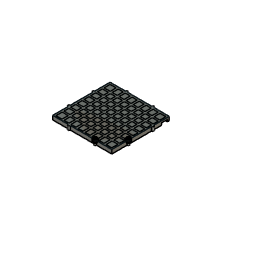
WS2812B_LED_Matrix_Diffuser (Autodesk Fusion 360 design; units mm, degrees)
Autodesk Fusion 360 part; units mm, degrees
note: some values were not read from the file. Set by a fixed rule: which face or edge a step refers to.
sketch "diffuser_base" plane through (0, 0, 0) normal (0, 0, 1) x (-1, 0, 0)
  circle A0 centre (-25.65, 24.4714) radius 1.425
  circle A1 centre (-0.15, 24.4714) radius 1.425
  circle A2 centre (25.35, 24.4714) radius 1.425
  circle A3 centre (-25.65, -24.5286) radius 1.425
  circle A4 centre (-0.15, -24.5286) radius 1.425
  circle A5 centre (25.35, -24.5286) radius 1.425
  line L0 (-33.5, -32.5) -> (-33.5, 32.5)
  line L1 (-33.5, 32.5) -> (33.5, 32.5)
  line L2 (33.5, 32.5) -> (33.5, -32.5)
  line L3 (33.5, -32.5) -> (-33.5, -32.5)
  line L4 (33.9, -32.9) -> (-33.9, -32.9)
  line L5 (-33.9, -32.9) -> (-33.9, 32.9)
  line L6 (-33.9, 32.9) -> (33.9, 32.9)
  line L7 (33.9, 32.9) -> (33.9, -32.9)
  line L8 (35.9, -34.9) -> (-35.9, -34.9)
  line L9 (-35.9, -34.9) -> (-35.9, 34.9)
  line L10 (-35.9, 34.9) -> (35.9, 34.9)
  line L11 (35.9, 34.9) -> (35.9, -34.9)
  dimension "d89" = -0.4
  dimension "d90" = -2.4
extrude "Extrude1" add sketch "diffuser_base" along normal blind 3.5 contours L8 L9 L10 L11
sketch "separations" plane through (0, 0, 1.5) normal (0, 0, 1) x (-1, 0, 0)
  circle A0 centre (25.35, 24.4714) radius 1.425
  circle A1 centre (-25.65, -24.5286) radius 1.425
  circle A2 centre (-0.15, -24.5286) radius 1.425
  circle A3 centre (25.35, -24.5286) radius 1.425
  line L0 (-27.4, 22.7571) -> (-27.4, 17.7571)
  line L1 (-27.4, 17.7571) -> (-32.4, 17.7571)
  line L2 (-32.4, 17.7571) -> (-32.4, 22.7571)
  line L3 (-32.4, 22.7571) -> (-27.4, 22.7571)
  line L4 (-18.9, 22.7571) -> (-18.9, 17.7571)
  line L5 (-18.9, 17.7571) -> (-23.9, 17.7571)
  line L6 (-23.9, 17.7571) -> (-23.9, 22.7571)
  line L7 (-23.9, 22.7571) -> (-18.9, 22.7571)
  line L8 (-10.4, 22.7571) -> (-10.4, 17.7571)
  line L9 (-10.4, 17.7571) -> (-15.4, 17.7571)
  line L10 (-15.4, 17.7571) -> (-15.4, 22.7571)
  line L11 (-15.4, 22.7571) -> (-10.4, 22.7571)
  line L12 (-1.9, 22.7571) -> (-1.9, 17.7571)
  line L13 (-1.9, 17.7571) -> (-6.9, 17.7571)
  line L14 (-6.9, 17.7571) -> (-6.9, 22.7571)
  line L15 (-6.9, 22.7571) -> (-1.9, 22.7571)
  line L16 (6.6, 22.7571) -> (6.6, 17.7571)
  line L17 (6.6, 17.7571) -> (1.6, 17.7571)
  line L18 (1.6, 17.7571) -> (1.6, 22.7571)
  line L19 (1.6, 22.7571) -> (6.6, 22.7571)
  line L20 (15.1, 22.7571) -> (15.1, 17.7571)
  line L21 (15.1, 17.7571) -> (10.1, 17.7571)
  line L22 (10.1, 17.7571) -> (10.1, 22.7571)
  line L23 (10.1, 22.7571) -> (15.1, 22.7571)
  line L24 (23.6, 22.7571) -> (23.6, 17.7571)
  line L25 (23.6, 17.7571) -> (18.6, 17.7571)
  line L26 (18.6, 17.7571) -> (18.6, 22.7571)
  line L27 (18.6, 22.7571) -> (23.6, 22.7571)
  line L28 (32.1, 22.7571) -> (32.1, 17.7571)
  line L29 (32.1, 17.7571) -> (27.1, 17.7571)
  line L30 (27.1, 17.7571) -> (27.1, 22.7571)
  line L31 (27.1, 22.7571) -> (32.1, 22.7571)
  line L32 (-27.4, 14.6143) -> (-27.4, 9.6143)
  line L33 (-27.4, 9.6143) -> (-32.4, 9.6143)
  line L34 (-32.4, 9.6143) -> (-32.4, 14.6143)
  line L35 (-32.4, 14.6143) -> (-27.4, 14.6143)
  line L36 (-18.9, 14.6143) -> (-18.9, 9.6143)
  line L37 (-18.9, 9.6143) -> (-23.9, 9.6143)
  line L38 (-23.9, 9.6143) -> (-23.9, 14.6143)
  line L39 (-23.9, 14.6143) -> (-18.9, 14.6143)
  line L40 (-10.4, 14.6143) -> (-10.4, 9.6143)
  line L41 (-10.4, 9.6143) -> (-15.4, 9.6143)
  line L42 (-15.4, 9.6143) -> (-15.4, 14.6143)
  line L43 (-15.4, 14.6143) -> (-10.4, 14.6143)
  line L44 (-1.9, 14.6143) -> (-1.9, 9.6143)
  line L45 (-1.9, 9.6143) -> (-6.9, 9.6143)
  line L46 (-6.9, 9.6143) -> (-6.9, 14.6143)
  line L47 (-6.9, 14.6143) -> (-1.9, 14.6143)
  line L48 (6.6, 14.6143) -> (6.6, 9.6143)
  line L49 (6.6, 9.6143) -> (1.6, 9.6143)
  line L50 (1.6, 9.6143) -> (1.6, 14.6143)
  line L51 (1.6, 14.6143) -> (6.6, 14.6143)
  line L52 (15.1, 14.6143) -> (15.1, 9.6143)
  line L53 (15.1, 9.6143) -> (10.1, 9.6143)
  line L54 (10.1, 9.6143) -> (10.1, 14.6143)
  line L55 (10.1, 14.6143) -> (15.1, 14.6143)
  line L56 (23.6, 14.6143) -> (23.6, 9.6143)
  line L57 (23.6, 9.6143) -> (18.6, 9.6143)
  line L58 (18.6, 9.6143) -> (18.6, 14.6143)
  line L59 (18.6, 14.6143) -> (23.6, 14.6143)
  line L60 (32.1, 14.6143) -> (32.1, 9.6143)
  line L61 (32.1, 9.6143) -> (27.1, 9.6143)
  line L62 (27.1, 9.6143) -> (27.1, 14.6143)
  line L63 (27.1, 14.6143) -> (32.1, 14.6143)
  line L64 (-27.4, 6.4714) -> (-27.4, 1.4714)
  line L65 (-27.4, 1.4714) -> (-32.4, 1.4714)
  line L66 (-32.4, 1.4714) -> (-32.4, 6.4714)
  line L67 (-32.4, 6.4714) -> (-27.4, 6.4714)
  line L68 (-18.9, 6.4714) -> (-18.9, 1.4714)
  line L69 (-18.9, 1.4714) -> (-23.9, 1.4714)
  line L70 (-23.9, 1.4714) -> (-23.9, 6.4714)
  line L71 (-23.9, 6.4714) -> (-18.9, 6.4714)
  line L72 (-10.4, 6.4714) -> (-10.4, 1.4714)
  line L73 (-10.4, 1.4714) -> (-15.4, 1.4714)
  line L74 (-15.4, 1.4714) -> (-15.4, 6.4714)
  line L75 (-15.4, 6.4714) -> (-10.4, 6.4714)
  line L76 (-1.9, 6.4714) -> (-1.9, 1.4714)
  line L77 (-1.9, 1.4714) -> (-6.9, 1.4714)
  line L78 (-6.9, 1.4714) -> (-6.9, 6.4714)
  line L79 (-6.9, 6.4714) -> (-1.9, 6.4714)
  line L80 (6.6, 6.4714) -> (6.6, 1.4714)
  line L81 (6.6, 1.4714) -> (1.6, 1.4714)
  line L82 (1.6, 1.4714) -> (1.6, 6.4714)
  line L83 (1.6, 6.4714) -> (6.6, 6.4714)
  line L84 (15.1, 6.4714) -> (15.1, 1.4714)
  line L85 (15.1, 1.4714) -> (10.1, 1.4714)
  line L86 (10.1, 1.4714) -> (10.1, 6.4714)
  line L87 (10.1, 6.4714) -> (15.1, 6.4714)
  line L88 (23.6, 6.4714) -> (23.6, 1.4714)
  line L89 (23.6, 1.4714) -> (18.6, 1.4714)
  line L90 (18.6, 1.4714) -> (18.6, 6.4714)
  line L91 (18.6, 6.4714) -> (23.6, 6.4714)
  line L92 (32.1, 6.4714) -> (32.1, 1.4714)
  line L93 (32.1, 1.4714) -> (27.1, 1.4714)
  line L94 (27.1, 1.4714) -> (27.1, 6.4714)
  line L95 (27.1, 6.4714) -> (32.1, 6.4714)
  line L96 (-27.4, -1.6714) -> (-27.4, -6.6714)
  line L97 (-27.4, -6.6714) -> (-32.4, -6.6714)
  line L98 (-32.4, -6.6714) -> (-32.4, -1.6714)
  line L99 (-32.4, -1.6714) -> (-27.4, -1.6714)
  line L100 (-18.9, -1.6714) -> (-18.9, -6.6714)
  line L101 (-18.9, -6.6714) -> (-23.9, -6.6714)
  line L102 (-23.9, -6.6714) -> (-23.9, -1.6714)
  line L103 (-23.9, -1.6714) -> (-18.9, -1.6714)
  line L104 (-10.4, -1.6714) -> (-10.4, -6.6714)
  line L105 (-10.4, -6.6714) -> (-15.4, -6.6714)
  line L106 (-15.4, -6.6714) -> (-15.4, -1.6714)
  line L107 (-15.4, -1.6714) -> (-10.4, -1.6714)
  line L108 (-1.9, -1.6714) -> (-1.9, -6.6714)
  line L109 (-1.9, -6.6714) -> (-6.9, -6.6714)
  line L110 (-6.9, -6.6714) -> (-6.9, -1.6714)
  line L111 (-6.9, -1.6714) -> (-1.9, -1.6714)
  line L112 (6.6, -1.6714) -> (6.6, -6.6714)
  line L113 (6.6, -6.6714) -> (1.6, -6.6714)
  line L114 (1.6, -6.6714) -> (1.6, -1.6714)
  line L115 (1.6, -1.6714) -> (6.6, -1.6714)
  line L116 (15.1, -1.6714) -> (15.1, -6.6714)
  line L117 (15.1, -6.6714) -> (10.1, -6.6714)
  line L118 (10.1, -6.6714) -> (10.1, -1.6714)
  line L119 (10.1, -1.6714) -> (15.1, -1.6714)
  line L120 (23.6, -1.6714) -> (23.6, -6.6714)
  line L121 (23.6, -6.6714) -> (18.6, -6.6714)
  line L122 (18.6, -6.6714) -> (18.6, -1.6714)
  line L123 (18.6, -1.6714) -> (23.6, -1.6714)
  line L124 (32.1, -1.6714) -> (32.1, -6.6714)
  line L125 (32.1, -6.6714) -> (27.1, -6.6714)
  line L126 (27.1, -6.6714) -> (27.1, -1.6714)
  line L127 (27.1, -1.6714) -> (32.1, -1.6714)
  line L128 (-27.4, -9.8143) -> (-27.4, -14.8143)
  line L129 (-27.4, -14.8143) -> (-32.4, -14.8143)
  line L130 (-32.4, -14.8143) -> (-32.4, -9.8143)
  line L131 (-32.4, -9.8143) -> (-27.4, -9.8143)
  line L132 (-18.9, -9.8143) -> (-18.9, -14.8143)
  line L133 (-18.9, -14.8143) -> (-23.9, -14.8143)
  line L134 (-23.9, -14.8143) -> (-23.9, -9.8143)
  line L135 (-23.9, -9.8143) -> (-18.9, -9.8143)
  line L136 (-10.4, -9.8143) -> (-10.4, -14.8143)
  line L137 (-10.4, -14.8143) -> (-15.4, -14.8143)
  line L138 (-15.4, -14.8143) -> (-15.4, -9.8143)
  line L139 (-15.4, -9.8143) -> (-10.4, -9.8143)
  line L140 (-1.9, -9.8143) -> (-1.9, -14.8143)
  line L141 (-1.9, -14.8143) -> (-6.9, -14.8143)
  line L142 (-6.9, -14.8143) -> (-6.9, -9.8143)
  line L143 (-6.9, -9.8143) -> (-1.9, -9.8143)
  line L144 (6.6, -9.8143) -> (6.6, -14.8143)
  line L145 (6.6, -14.8143) -> (1.6, -14.8143)
  line L146 (1.6, -14.8143) -> (1.6, -9.8143)
  line L147 (1.6, -9.8143) -> (6.6, -9.8143)
  line L148 (15.1, -9.8143) -> (15.1, -14.8143)
  line L149 (15.1, -14.8143) -> (10.1, -14.8143)
  line L150 (10.1, -14.8143) -> (10.1, -9.8143)
  line L151 (10.1, -9.8143) -> (15.1, -9.8143)
  line L152 (23.6, -9.8143) -> (23.6, -14.8143)
  line L153 (23.6, -14.8143) -> (18.6, -14.8143)
  line L154 (18.6, -14.8143) -> (18.6, -9.8143)
  line L155 (18.6, -9.8143) -> (23.6, -9.8143)
  line L156 (32.1, -9.8143) -> (32.1, -14.8143)
  line L157 (32.1, -14.8143) -> (27.1, -14.8143)
  line L158 (27.1, -14.8143) -> (27.1, -9.8143)
  line L159 (27.1, -9.8143) -> (32.1, -9.8143)
  line L160 (-27.4, -17.9571) -> (-27.4, -22.9571)
  line L161 (-27.4, -22.9571) -> (-32.4, -22.9571)
  line L162 (-32.4, -22.9571) -> (-32.4, -17.9571)
  line L163 (-32.4, -17.9571) -> (-27.4, -17.9571)
  line L164 (-18.9, -17.9571) -> (-18.9, -22.9571)
  line L165 (-18.9, -22.9571) -> (-23.9, -22.9571)
  line L166 (-23.9, -22.9571) -> (-23.9, -17.9571)
  line L167 (-23.9, -17.9571) -> (-18.9, -17.9571)
  line L168 (-10.4, -17.9571) -> (-10.4, -22.9571)
  line L169 (-10.4, -22.9571) -> (-15.4, -22.9571)
  line L170 (-15.4, -22.9571) -> (-15.4, -17.9571)
  line L171 (-15.4, -17.9571) -> (-10.4, -17.9571)
  line L172 (-1.9, -17.9571) -> (-1.9, -22.9571)
  line L173 (-1.9, -22.9571) -> (-6.9, -22.9571)
  line L174 (-6.9, -22.9571) -> (-6.9, -17.9571)
  line L175 (-6.9, -17.9571) -> (-1.9, -17.9571)
  line L176 (6.6, -17.9571) -> (6.6, -22.9571)
  line L177 (6.6, -22.9571) -> (1.6, -22.9571)
  line L178 (1.6, -22.9571) -> (1.6, -17.9571)
  line L179 (1.6, -17.9571) -> (6.6, -17.9571)
  line L180 (15.1, -17.9571) -> (15.1, -22.9571)
  line L181 (15.1, -22.9571) -> (10.1, -22.9571)
  line L182 (10.1, -22.9571) -> (10.1, -17.9571)
  line L183 (10.1, -17.9571) -> (15.1, -17.9571)
  line L184 (23.6, -17.9571) -> (23.6, -22.9571)
  line L185 (23.6, -22.9571) -> (18.6, -22.9571)
  line L186 (18.6, -22.9571) -> (18.6, -17.9571)
  line L187 (18.6, -17.9571) -> (23.6, -17.9571)
  line L188 (32.1, -17.9571) -> (32.1, -22.9571)
  line L189 (32.1, -22.9571) -> (27.1, -22.9571)
  line L190 (27.1, -22.9571) -> (27.1, -17.9571)
  line L191 (27.1, -17.9571) -> (32.1, -17.9571)
  line L192 (-27.4, -26.1) -> (-27.4, -31.1)
  line L193 (-27.4, -31.1) -> (-32.4, -31.1)
  line L194 (-32.4, -31.1) -> (-32.4, -26.1)
  line L195 (-32.4, -26.1) -> (-27.4, -26.1)
  line L196 (-18.9, -26.1) -> (-18.9, -31.1)
  line L197 (-18.9, -31.1) -> (-23.9, -31.1)
  line L198 (-23.9, -31.1) -> (-23.9, -26.1)
  line L199 (-23.9, -26.1) -> (-18.9, -26.1)
  line L200 (-10.4, -26.1) -> (-10.4, -31.1)
  line L201 (-10.4, -31.1) -> (-15.4, -31.1)
  line L202 (-15.4, -31.1) -> (-15.4, -26.1)
  line L203 (-15.4, -26.1) -> (-10.4, -26.1)
  line L204 (-1.9, -26.1) -> (-1.9, -31.1)
  line L205 (-1.9, -31.1) -> (-6.9, -31.1)
  line L206 (-6.9, -31.1) -> (-6.9, -26.1)
  line L207 (-6.9, -26.1) -> (-1.9, -26.1)
  line L208 (6.6, -26.1) -> (6.6, -31.1)
  line L209 (6.6, -31.1) -> (1.6, -31.1)
  line L210 (1.6, -31.1) -> (1.6, -26.1)
  line L211 (1.6, -26.1) -> (6.6, -26.1)
  line L212 (15.1, -26.1) -> (15.1, -31.1)
  line L213 (15.1, -31.1) -> (10.1, -31.1)
  line L214 (10.1, -31.1) -> (10.1, -26.1)
  line L215 (10.1, -26.1) -> (15.1, -26.1)
  line L216 (23.6, -26.1) -> (23.6, -31.1)
  line L217 (23.6, -31.1) -> (18.6, -31.1)
  line L218 (18.6, -31.1) -> (18.6, -26.1)
  line L219 (18.6, -26.1) -> (23.6, -26.1)
  line L220 (32.1, -26.1) -> (32.1, -31.1)
  line L221 (32.1, -31.1) -> (27.1, -31.1)
  line L222 (27.1, -31.1) -> (27.1, -26.1)
  line L223 (27.1, -26.1) -> (32.1, -26.1)
  line L224 (-33.5, 32.5) -> (-33.5, -32.5)
  line L225 (-33.5, -32.5) -> (33.5, -32.5)
  line L226 (33.5, -32.5) -> (33.5, 32.5)
  line L227 (33.5, 32.5) -> (-33.5, 32.5)
  line L228 (-27.4, -26.1) -> (-32.4, -26.1)
  line L229 (-32.4, -22.9571) -> (-27.4, -22.9571)
  line L230 (33.9, -25.6) -> (-33.9, -25.6)
  line L231 (-33.9, -25.6) -> (-33.9, -23.4571)
  line L232 (-33.9, -23.4571) -> (33.9, -23.4571)
  line L233 (33.9, -23.4571) -> (33.9, -25.6)
  line L234 (-23.9, -26.1) -> (-23.9, -31.1)
  line L235 (-27.4, -31.1) -> (-27.4, -26.1)
  line L236 (-24.4, -32.9) -> (-26.9, -32.9)
  line L237 (-26.9, -32.9) -> (-26.9, 32.9)
  line L238 (-26.9, 32.9) -> (-24.4, 32.9)
  line L239 (-24.4, 32.9) -> (-24.4, -32.9)
  circle A4 centre (-25.65, 24.4714) radius 1.425
  circle A5 centre (-0.15, 24.4714) radius 1.425
  line L240 (-27.4, 30.9) -> (-27.4, 25.9)
  line L241 (-27.4, 25.9) -> (-32.4, 25.9)
  line L242 (-32.4, 25.9) -> (-32.4, 30.9)
  line L243 (-32.4, 30.9) -> (-27.4, 30.9)
  line L244 (-18.9, 30.9) -> (-18.9, 25.9)
  line L245 (-18.9, 25.9) -> (-23.9, 25.9)
  line L246 (-23.9, 25.9) -> (-23.9, 30.9)
  line L247 (-23.9, 30.9) -> (-18.9, 30.9)
  line L248 (-10.4, 30.9) -> (-10.4, 25.9)
  line L249 (-10.4, 25.9) -> (-15.4, 25.9)
  line L250 (-15.4, 25.9) -> (-15.4, 30.9)
  line L251 (-15.4, 30.9) -> (-10.4, 30.9)
  line L252 (-1.9, 30.9) -> (-1.9, 25.9)
  line L253 (-1.9, 25.9) -> (-6.9, 25.9)
  line L254 (-6.9, 25.9) -> (-6.9, 30.9)
  line L255 (-6.9, 30.9) -> (-1.9, 30.9)
  line L256 (6.6, 30.9) -> (6.6, 25.9)
  line L257 (6.6, 25.9) -> (1.6, 25.9)
  line L258 (1.6, 25.9) -> (1.6, 30.9)
  line L259 (1.6, 30.9) -> (6.6, 30.9)
  line L260 (15.1, 30.9) -> (15.1, 25.9)
  line L261 (15.1, 25.9) -> (10.1, 25.9)
  line L262 (10.1, 25.9) -> (10.1, 30.9)
  line L263 (10.1, 30.9) -> (15.1, 30.9)
  line L264 (23.6, 30.9) -> (23.6, 25.9)
  line L265 (23.6, 25.9) -> (18.6, 25.9)
  line L266 (18.6, 25.9) -> (18.6, 30.9)
  line L267 (18.6, 30.9) -> (23.6, 30.9)
  line L268 (32.1, 30.9) -> (32.1, 25.9)
  line L269 (32.1, 25.9) -> (27.1, 25.9)
  line L270 (27.1, 25.9) -> (27.1, 30.9)
  line L271 (27.1, 30.9) -> (32.1, 30.9)
  line L272 (33.9, 32.9) -> (33.9, -32.9)
  line L273 (33.9, -32.9) -> (-33.9, -32.9)
  line L274 (-33.9, -32.9) -> (-33.9, 32.9)
  line L275 (-33.9, 32.9) -> (33.9, 32.9)
  dimension "d26" = 0.5
  dimension "d27" = 0.5
  dimension "d28" = 0.5
  dimension "d29" = 0.5
  constraint horizontal L230
  constraint vertical L231
  constraint horizontal L232
  constraint vertical L233
  constraint horizontal L236
  constraint vertical L237
  constraint horizontal L238
  constraint vertical L239
  constraint collinear L233 L272
  constraint collinear L231 L274
  constraint collinear L236 L273
  constraint collinear L238 L275
  measures "d26" distance of L228 L230
  measures "d27" distance of L229 L232
  measures "d28" distance of L234 L239
  measures "d29" distance of L235 L237
extrude "Extrude2" add sketch "separations" along normal blind 2 contours A1 L230 L232 L237 L239 | A1 L232 L239 | A1 L230 L239 | A1 L232 | A1 L232 L237 L239 A4 | A1 L225 L230 L237 L239 | A1 L230 | A1 L232 L237 | L237 L239 A4 | A1 L230 L237 | L225 L236 L237 L239 L273 | L227 L237 L239 A4 | L227 L237 L238 L239 L275
extrude "Extrude3" add sketch "separations" along normal blind 2 contours A1 L239 | A1 A2 L230 L232 L239 | A2 L230 L232 | A1 L237 | A1 L224 L230 L232 L237 | A2 A3 L230 L232 | L224 L230 L231 L232 L274 | A3 L230 L232 | A3 L226 L230 L232 | L226 L230 L232 L233 L272
pattern_linear "R-Pattern1" count 7 spacing 8.5 along (-1, 0, 0) of "Extrude2"
pattern_linear "R-Pattern2" count 7 spacing 8.15 along (0, -1, 0) of "Extrude3"
sketch "cover" plane through (0, 0, 3.5) normal (0, 0, 1) x (-1, 0, 0)
  line L0 (-26.9, 32.9) -> (-26.9, 25.4429)
  line L1 (-26.9, 25.4429) -> (-33.9, 25.4429)
  line L2 (33.9, 17.2929) -> (26.6, 17.2929)
  line L3 (26.6, 17.2929) -> (26.6, 23.3)
  line L4 (26.6, 23.3) -> (33.9, 23.3)
  line L5 (18.1, 25.4429) -> (18.1, 32.9)
  line L6 (24.1, 32.9) -> (24.1, 25.4429)
  line L7 (24.1, 25.4429) -> (18.1, 25.4429)
  line L8 (15.6, 23.3) -> (15.6, 17.2929)
  line L9 (15.6, 17.2929) -> (9.6, 17.2929)
  line L10 (9.6, 17.2929) -> (9.6, 23.3)
  line L11 (9.6, 23.3) -> (15.6, 23.3)
  line L12 (7.1, 23.3) -> (7.1, 17.2929)
  line L13 (7.1, 17.2929) -> (1.1, 17.2929)
  line L14 (1.1, 17.2929) -> (1.1, 23.3)
  line L15 (1.1, 23.3) -> (7.1, 23.3)
  line L16 (-1.4, 23.3) -> (-1.4, 17.2929)
  line L17 (-1.4, 17.2929) -> (-7.4, 17.2929)
  line L18 (-7.4, 17.2929) -> (-7.4, 23.3)
  line L19 (-7.4, 23.3) -> (-1.4, 23.3)
  line L20 (-9.9, 23.3) -> (-9.9, 17.2929)
  line L21 (-9.9, 17.2929) -> (-15.9, 17.2929)
  line L22 (-15.9, 17.2929) -> (-15.9, 23.3)
  line L23 (-15.9, 23.3) -> (-9.9, 23.3)
  line L24 (-18.4, 23.3) -> (-18.4, 17.2929)
  line L25 (-18.4, 17.2929) -> (-24.4, 17.2929)
  line L26 (-24.4, 17.2929) -> (-24.4, 23.3)
  line L27 (-24.4, 23.3) -> (-18.4, 23.3)
  line L28 (18.1, 23.3) -> (24.1, 23.3)
  line L29 (24.1, 23.3) -> (24.1, 17.2929)
  line L30 (24.1, 17.2929) -> (18.1, 17.2929)
  line L31 (18.1, 17.2929) -> (18.1, 23.3)
  line L32 (15.6, 25.4429) -> (9.6, 25.4429)
  line L33 (9.6, 25.4429) -> (9.6, 32.9)
  line L34 (7.1, 25.4429) -> (1.1, 25.4429)
  line L35 (1.1, 25.4429) -> (1.1, 32.9)
  line L36 (-1.4, 25.4429) -> (-7.4, 25.4429)
  line L37 (-7.4, 25.4429) -> (-7.4, 32.9)
  line L38 (-9.9, 25.4429) -> (-15.9, 25.4429)
  line L39 (-15.9, 25.4429) -> (-15.9, 32.9)
  line L40 (26.6, 25.4429) -> (26.6, 32.9)
  line L41 (-18.4, 25.4429) -> (-24.4, 25.4429)
  line L42 (-24.4, 25.4429) -> (-24.4, 32.9)
  line L43 (-33.9, 23.3) -> (-26.9, 23.3)
  line L44 (-26.9, 23.3) -> (-26.9, 17.2929)
  line L45 (-26.9, 17.2929) -> (-33.9, 17.2929)
  line L46 (33.9, 9.1429) -> (26.6, 9.1429)
  line L47 (26.6, 9.1429) -> (26.6, 15.15)
  line L48 (26.6, 15.15) -> (33.9, 15.15)
  line L49 (24.1, 15.15) -> (24.1, 9.1429)
  line L50 (24.1, 9.1429) -> (18.1, 9.1429)
  line L51 (18.1, 9.1429) -> (18.1, 15.15)
  line L52 (18.1, 15.15) -> (24.1, 15.15)
  line L53 (15.6, 15.15) -> (15.6, 9.1429)
  line L54 (15.6, 9.1429) -> (9.6, 9.1429)
  line L55 (9.6, 9.1429) -> (9.6, 15.15)
  line L56 (9.6, 15.15) -> (15.6, 15.15)
  line L57 (7.1, 15.15) -> (7.1, 9.1429)
  line L58 (7.1, 9.1429) -> (1.1, 9.1429)
  line L59 (1.1, 9.1429) -> (1.1, 15.15)
  line L60 (1.1, 15.15) -> (7.1, 15.15)
  line L61 (-1.4, 15.15) -> (-1.4, 9.1429)
  line L62 (-1.4, 9.1429) -> (-7.4, 9.1429)
  line L63 (-7.4, 9.1429) -> (-7.4, 15.15)
  line L64 (-7.4, 15.15) -> (-1.4, 15.15)
  line L65 (-9.9, 15.15) -> (-9.9, 9.1429)
  line L66 (-9.9, 9.1429) -> (-15.9, 9.1429)
  line L67 (-15.9, 9.1429) -> (-15.9, 15.15)
  line L68 (-15.9, 15.15) -> (-9.9, 15.15)
  line L69 (-18.4, 15.15) -> (-18.4, 9.1429)
  line L70 (-18.4, 9.1429) -> (-24.4, 9.1429)
  line L71 (-24.4, 9.1429) -> (-24.4, 15.15)
  line L72 (-24.4, 15.15) -> (-18.4, 15.15)
  line L73 (-33.9, 7) -> (-26.9, 7)
  line L74 (-26.9, 7) -> (-26.9, 0.9929)
  line L75 (-26.9, 0.9929) -> (-33.9, 0.9929)
  line L76 (33.9, -7.1571) -> (26.6, -7.1571)
  line L77 (26.6, -7.1571) -> (26.6, -1.15)
  line L78 (26.6, -1.15) -> (33.9, -1.15)
  line L79 (24.1, -1.15) -> (24.1, -7.1571)
  line L80 (24.1, -7.1571) -> (18.1, -7.1571)
  line L81 (18.1, -7.1571) -> (18.1, -1.15)
  line L82 (18.1, -1.15) -> (24.1, -1.15)
  line L83 (-18.4, -1.15) -> (-18.4, -7.1571)
  line L84 (-18.4, -7.1571) -> (-24.4, -7.1571)
  line L85 (-24.4, -7.1571) -> (-24.4, -1.15)
  line L86 (-24.4, -1.15) -> (-18.4, -1.15)
  line L87 (-15.9, -1.15) -> (-9.9, -1.15)
  line L88 (-9.9, -1.15) -> (-9.9, -7.1571)
  line L89 (-9.9, -7.1571) -> (-15.9, -7.1571)
  line L90 (-15.9, -7.1571) -> (-15.9, -1.15)
  line L91 (-7.4, -1.15) -> (-1.4, -1.15)
  line L92 (-1.4, -1.15) -> (-1.4, -7.1571)
  line L93 (-1.4, -7.1571) -> (-7.4, -7.1571)
  line L94 (-7.4, -7.1571) -> (-7.4, -1.15)
  line L95 (1.1, -1.15) -> (7.1, -1.15)
  line L96 (7.1, -1.15) -> (7.1, -7.1571)
  line L97 (7.1, -7.1571) -> (1.1, -7.1571)
  line L98 (1.1, -7.1571) -> (1.1, -1.15)
  line L99 (9.6, -1.15) -> (15.6, -1.15)
  line L100 (15.6, -1.15) -> (15.6, -7.1571)
  line L101 (15.6, -7.1571) -> (9.6, -7.1571)
  line L102 (9.6, -7.1571) -> (9.6, -1.15)
  line L103 (-33.9, -1.15) -> (-26.9, -1.15)
  line L104 (-26.9, -1.15) -> (-26.9, -7.1571)
  line L105 (-26.9, -7.1571) -> (-33.9, -7.1571)
  line L106 (33.9, -15.3071) -> (26.6, -15.3071)
  line L107 (26.6, -15.3071) -> (26.6, -9.3)
  line L108 (26.6, -9.3) -> (33.9, -9.3)
  line L109 (7.1, -9.3) -> (7.1, -15.3071)
  line L110 (7.1, -15.3071) -> (1.1, -15.3071)
  line L111 (1.1, -15.3071) -> (1.1, -9.3)
  line L112 (1.1, -9.3) -> (7.1, -9.3)
  line L113 (-1.4, -9.3) -> (-1.4, -15.3071)
  line L114 (-1.4, -15.3071) -> (-7.4, -15.3071)
  line L115 (-7.4, -15.3071) -> (-7.4, -9.3)
  line L116 (-7.4, -9.3) -> (-1.4, -9.3)
  line L117 (-18.4, -9.3) -> (-18.4, -15.3071)
  line L118 (-18.4, -15.3071) -> (-24.4, -15.3071)
  line L119 (-24.4, -15.3071) -> (-24.4, -9.3)
  line L120 (-24.4, -9.3) -> (-18.4, -9.3)
  line L121 (24.1, -9.3) -> (24.1, -15.3071)
  line L122 (24.1, -15.3071) -> (18.1, -15.3071)
  line L123 (18.1, -15.3071) -> (18.1, -9.3)
  line L124 (18.1, -9.3) -> (24.1, -9.3)
  line L125 (9.6, -9.3) -> (15.6, -9.3)
  line L126 (15.6, -9.3) -> (15.6, -15.3071)
  line L127 (15.6, -15.3071) -> (9.6, -15.3071)
  line L128 (9.6, -15.3071) -> (9.6, -9.3)
  line L129 (-15.9, -9.3) -> (-9.9, -9.3)
  line L130 (-9.9, -9.3) -> (-9.9, -15.3071)
  line L131 (-9.9, -15.3071) -> (-15.9, -15.3071)
  line L132 (-15.9, -15.3071) -> (-15.9, -9.3)
  line L133 (-33.9, -9.3) -> (-26.9, -9.3)
  line L134 (-26.9, -9.3) -> (-26.9, -15.3071)
  line L135 (-26.9, -15.3071) -> (-33.9, -15.3071)
  line L136 (33.9, -23.4571) -> (26.6, -23.4571)
  line L137 (26.6, -23.4571) -> (26.6, -17.45)
  line L138 (26.6, -17.45) -> (33.9, -17.45)
  line L139 (24.1, -17.45) -> (24.1, -23.4571)
  line L140 (24.1, -23.4571) -> (18.1, -23.4571)
  line L141 (18.1, -23.4571) -> (18.1, -17.45)
  line L142 (18.1, -17.45) -> (24.1, -17.45)
  line L143 (15.6, -17.45) -> (15.6, -23.4571)
  line L144 (15.6, -23.4571) -> (9.6, -23.4571)
  line L145 (9.6, -23.4571) -> (9.6, -17.45)
  line L146 (9.6, -17.45) -> (15.6, -17.45)
  line L147 (7.1, -17.45) -> (7.1, -23.4571)
  line L148 (7.1, -23.4571) -> (1.1, -23.4571)
  line L149 (1.1, -23.4571) -> (1.1, -17.45)
  line L150 (1.1, -17.45) -> (7.1, -17.45)
  line L151 (-1.4, -17.45) -> (-1.4, -23.4571)
  line L152 (-1.4, -23.4571) -> (-7.4, -23.4571)
  line L153 (-7.4, -23.4571) -> (-7.4, -17.45)
  line L154 (-7.4, -17.45) -> (-1.4, -17.45)
  line L155 (-18.4, -17.45) -> (-18.4, -23.4571)
  line L156 (-18.4, -23.4571) -> (-24.4, -23.4571)
  line L157 (-24.4, -23.4571) -> (-24.4, -17.45)
  line L158 (-24.4, -17.45) -> (-18.4, -17.45)
  line L159 (-15.9, -17.45) -> (-9.9, -17.45)
  line L160 (-9.9, -17.45) -> (-9.9, -23.4571)
  line L161 (-9.9, -23.4571) -> (-15.9, -23.4571)
  line L162 (-15.9, -23.4571) -> (-15.9, -17.45)
  line L163 (1.1, -25.6) -> (7.1, -25.6)
  line L164 (7.1, -25.6) -> (7.1, -32.9)
  line L165 (-7.4, -25.6) -> (-1.4, -25.6)
  line L166 (-1.4, -25.6) -> (-1.4, -32.9)
  line L167 (-15.9, -25.6) -> (-9.9, -25.6)
  line L168 (-9.9, -25.6) -> (-9.9, -32.9)
  line L169 (-24.4, -25.6) -> (-18.4, -25.6)
  line L170 (-18.4, -25.6) -> (-18.4, -32.9)
  line L171 (-33.9, -25.6) -> (-26.9, -25.6)
  line L172 (-26.9, -25.6) -> (-26.9, -32.9)
  line L173 (-33.9, -17.45) -> (-26.9, -17.45)
  line L174 (-26.9, -17.45) -> (-26.9, -23.4571)
  line L175 (-26.9, -23.4571) -> (-33.9, -23.4571)
  line L176 (9.6, -25.6) -> (15.6, -25.6)
  line L177 (15.6, -25.6) -> (15.6, -32.9)
  line L178 (26.6, -25.6) -> (33.9, -25.6)
  line L179 (18.1, -25.6) -> (24.1, -25.6)
  line L180 (24.1, -25.6) -> (24.1, -32.9)
  line L181 (18.1, 7) -> (24.1, 7)
  line L182 (24.1, 7) -> (24.1, 0.9929)
  line L183 (24.1, 0.9929) -> (18.1, 0.9929)
  line L184 (18.1, 0.9929) -> (18.1, 7)
  line L185 (9.6, 7) -> (15.6, 7)
  line L186 (15.6, 7) -> (15.6, 0.9929)
  line L187 (15.6, 0.9929) -> (9.6, 0.9929)
  line L188 (9.6, 0.9929) -> (9.6, 7)
  line L189 (1.1, 7) -> (7.1, 7)
  line L190 (7.1, 7) -> (7.1, 0.9929)
  line L191 (7.1, 0.9929) -> (1.1, 0.9929)
  line L192 (1.1, 0.9929) -> (1.1, 7)
  line L193 (-7.4, 7) -> (-1.4, 7)
  line L194 (-1.4, 7) -> (-1.4, 0.9929)
  line L195 (-1.4, 0.9929) -> (-7.4, 0.9929)
  line L196 (-7.4, 0.9929) -> (-7.4, 7)
  line L197 (-15.9, 7) -> (-9.9, 7)
  line L198 (-9.9, 7) -> (-9.9, 0.9929)
  line L199 (-9.9, 0.9929) -> (-15.9, 0.9929)
  line L200 (-15.9, 0.9929) -> (-15.9, 7)
  line L201 (-18.4, 7) -> (-18.4, 0.9929)
  line L202 (-18.4, 0.9929) -> (-24.4, 0.9929)
  line L203 (-24.4, 0.9929) -> (-24.4, 7)
  line L204 (-24.4, 7) -> (-18.4, 7)
  line L205 (26.6, 0.9929) -> (26.6, 7)
  line L206 (26.6, 7) -> (33.9, 7)
  line L207 (-33.9, 15.15) -> (-26.9, 15.15)
  line L208 (-26.9, 15.15) -> (-26.9, 9.1429)
  line L209 (-26.9, 9.1429) -> (-33.9, 9.1429)
  circle A0 centre (25.35, -24.5286) radius 1.425
  circle A1 centre (-0.15, -24.5286) radius 1.425
  circle A2 centre (-25.65, -24.5286) radius 1.425
  circle A3 centre (25.35, 24.4714) radius 1.425
  circle A4 centre (-0.15, 24.4714) radius 1.425
  circle A5 centre (-25.65, 24.4714) radius 1.425
  line L210 (18.1, 32.9) -> (24.1, 32.9)
  line L211 (9.6, 32.9) -> (15.6, 32.9)
  line L212 (15.6, 32.9) -> (15.6, 25.4429)
  line L213 (1.1, 32.9) -> (7.1, 32.9)
  line L214 (7.1, 32.9) -> (7.1, 25.4429)
  line L215 (-7.4, 32.9) -> (-1.4, 32.9)
  line L216 (-1.4, 32.9) -> (-1.4, 25.4429)
  line L217 (-15.9, 32.9) -> (-9.9, 32.9)
  line L218 (-9.9, 32.9) -> (-9.9, 25.4429)
  line L219 (26.6, 32.9) -> (33.9, 32.9)
  line L220 (33.9, 23.3) -> (33.9, 17.2929)
  line L221 (33.9, -32.9) -> (26.6, -32.9)
  line L222 (-24.4, 32.9) -> (-18.4, 32.9)
  line L223 (-18.4, 32.9) -> (-18.4, 25.4429)
  line L224 (15.6, -32.9) -> (9.6, -32.9)
  line L225 (9.6, -32.9) -> (9.6, -25.6)
  line L226 (-1.4, -32.9) -> (-7.4, -32.9)
  line L227 (-7.4, -32.9) -> (-7.4, -25.6)
  line L228 (-18.4, -32.9) -> (-24.4, -32.9)
  line L229 (-24.4, -32.9) -> (-24.4, -25.6)
  line L230 (35.9, 34.9) -> (-35.9, 34.9)
  line L231 (-35.9, 34.9) -> (-35.9, -34.9)
  line L232 (-35.9, -34.9) -> (35.9, -34.9)
  line L233 (35.9, -34.9) -> (35.9, 34.9)
  line L234 (-26.9, -32.9) -> (-33.9, -32.9)
  line L235 (-33.9, 25.4429) -> (-33.9, 32.9)
  line L236 (-33.9, 32.9) -> (-26.9, 32.9)
  line L237 (-9.9, -32.9) -> (-15.9, -32.9)
  line L238 (-15.9, -32.9) -> (-15.9, -25.6)
  line L239 (7.1, -32.9) -> (1.1, -32.9)
  line L240 (1.1, -32.9) -> (1.1, -25.6)
  line L241 (24.1, -32.9) -> (18.1, -32.9)
  line L242 (18.1, -32.9) -> (18.1, -25.6)
  line L243 (33.9, 25.4429) -> (26.6, 25.4429)
  line L244 (33.9, 32.9) -> (33.9, 25.4429)
  line L245 (-33.9, 17.2929) -> (-33.9, 23.3)
  line L246 (33.9, 15.15) -> (33.9, 9.1429)
  line L247 (-33.9, 0.9929) -> (-33.9, 7)
  line L248 (33.9, -1.15) -> (33.9, -7.1571)
  line L249 (-33.9, -7.1571) -> (-33.9, -1.15)
  line L250 (33.9, -9.3) -> (33.9, -15.3071)
  line L251 (-33.9, -15.3071) -> (-33.9, -9.3)
  line L252 (33.9, -17.45) -> (33.9, -23.4571)
  line L253 (-33.9, -32.9) -> (-33.9, -25.6)
  line L254 (-33.9, -23.4571) -> (-33.9, -17.45)
  line L255 (26.6, -32.9) -> (26.6, -25.6)
  line L256 (33.9, -25.6) -> (33.9, -32.9)
  line L257 (33.9, 7) -> (33.9, 0.9929)
  line L258 (33.9, 0.9929) -> (26.6, 0.9929)
  line L259 (-33.9, 9.1429) -> (-33.9, 15.15)
extrude "Extrude4" add sketch "cover" along normal blind 0.3 contours L0 L1 L235 L236 | L2 L3 L4 L220 | L5 L6 L7 L210 | L8 L9 L10 L11 | L12 L13 L14 L15 | L16 L17 L18 L19 | L20 L21 L22 L23 | L24 L25 L26 L27 | L28 L29 L30 L31 | L32 L33 L211 L212 | L34 L35 L213 L214 | L36 L37 L215 L216 | L38 L39 L217 L218 | L40 L219 L243 L244 | L41 L42 L222 L223 | L43 L44 L45 L245 | L46 L47 L48 L246 | L49 L50 L51 L52 | L53 L54 L55 L56 | L57 L58 L59 L60 | L61 L62 L63 L64 | L65 L66 L67 L68 | L69 L70 L71 L72 | L73 L74 L75 L247 | L76 L77 L78 L248 | L79 L80 L81 L82 | L83 L84 L85 L86 | L87 L88 L89 L90 | L91 L92 L93 L94 | L95 L96 L97 L98 | L99 L100 L101 L102 | L103 L104 L105 L249 | L106 L107 L108 L250 | L109 L110 L111 L112 | L113 L114 L115 L116 | L117 L118 L119 L120 | L121 L122 L123 L124 | L125 L126 L127 L128 | L129 L130 L131 L132 | L133 L134 L135 L251 | L136 L137 L138 L252 | L139 L140 L141 L142 | L143 L144 L145 L146 | L147 L148 L149 L150 | L151 L152 L153 L154 | L155 L156 L157 L158 | L159 L160 L161 L162 | L163 L164 L239 L240 | L165 L166 L226 L227 | L167 L168 L237 L238 | L169 L170 L228 L229 | L171 L172 L234 L253 | L173 L174 L175 L254 | L176 L177 L224 L225 | L178 L221 L255 L256 | L179 L180 L241 L242 | L181 L182 L183 L184 | L185 L186 L187 L188 | L189 L190 L191 L192 | L193 L194 L195 L196 | L197 L198 L199 L200 | L201 L202 L203 L204 | L205 L206 L257 L258 | L207 L208 L209 L259 | A0 | A1 | A2 | A3 | A4 | A5 | L230 L231 L232 L233
sketch "mounts" plane through (0, 0, 3.8) normal (0, 0, 1) x (-1, 0, 0)
  circle A0 centre (25.35, -24.5286) radius 1.425
  line L0 (35.9, -34.9) -> (35.9, 34.9)
  line L1 (35.9, 34.9) -> (-35.9, 34.9)
  line L2 (-35.9, 34.9) -> (-35.9, -34.9)
  line L3 (-35.9, -34.9) -> (35.9, -34.9)
  circle A1 centre (-0.15, -24.5286) radius 1.425
  circle A2 centre (-25.65, -24.5286) radius 1.425
  circle A3 centre (-25.65, 24.4714) radius 1.425
  circle A4 centre (-0.15, 24.4714) radius 1.425
  circle A5 centre (25.35, 24.4714) radius 1.425
extrude "Extrude5" add sketch "mounts" against normal blind 3.8 contours A0 | A1 | A2 | A3 | A4 | A5
extrude "Extrude6" add 1 faces at (11.3, 34.2333, 0) along direction (0, 0, -1) blind 1
extrude "Extrude15" add 25 faces at (-0.2692, 24.2055, 0) (25.319, -24.3314, 0) (25.319, 24.6686, 0) (-0.2692, -24.7945, 0) (-25.681, 24.6686, 0) (-25.7583, -23.993, 0) (-0.2692, 24.2055, 0) (25.319, -24.3314, 0) (25.319, 24.6686, 0) (-0.2692, -24.7945, 0) (-25.681, 24.6686, 0) (-25.7583, -23.993, 0) (-25.681, 24.6686, 0) (-0.2692, 24.2055, 0) (25.319, -24.3314, 0) (25.319, 24.6686, 0) (-0.2692, -24.7945, 0) (-25.681, 24.6686, 0) (-25.7583, -23.993, 0) (-0.2692, 24.2055, 0) (25.319, -24.3314, 0) (25.319, 24.6686, 0) (-0.2692, -24.7945, 0) (-25.681, 24.6686, 0) (-25.7583, -23.993, 0) along direction (0, 0, -1) blind 1
sketch "Sketch9" plane through (35.9, 0, 0) normal (1, 0, 0) x (0, 1, 0)
  line L0 (34.9, 3.5) -> (34.9, 3.8)
  line L1 (34.9, 3.8) -> (-34.9, 3.8)
  line L2 (-34.9, 3.8) -> (-34.9, 3.5)
  line L3 (32.9, -1) -> (25.6, -1)
  line L4 (25.6, -1) -> (25.6, 1.5)
  line L5 (25.6, 1.5) -> (32.9, 1.5)
  line L6 (32.9, 1.5) -> (32.9, -1)
  line L7 (-34.9, 3.5) -> (34.9, 3.5)
  line L8 (-25.4429, 3.5) -> (-25.4429, 1.5)
  line L9 (-25.4429, 1.5) -> (-23.3, 1.5)
  line L10 (-23.3, 1.5) -> (-23.3, 3.5)
  line L11 (-23.3, 3.5) -> (-17.2929, 3.5)
  line L12 (-17.2929, 3.5) -> (-17.2929, 1.5)
  line L13 (-17.2929, 1.5) -> (-15.15, 1.5)
  line L14 (-15.15, 1.5) -> (-15.15, 3.5)
  line L15 (-15.15, 3.5) -> (-9.1429, 3.5)
  line L16 (-9.1429, 3.5) -> (-9.1429, 1.5)
  line L17 (-9.1429, 1.5) -> (-7, 1.5)
  line L18 (-7, 1.5) -> (-7, 3.5)
  line L19 (-7, 3.5) -> (-0.9929, 3.5)
  line L20 (-0.9929, 3.5) -> (-0.9929, 1.5)
  line L21 (-0.9929, 1.5) -> (1.15, 1.5)
  line L22 (1.15, 1.5) -> (1.15, 3.5)
  line L23 (1.15, 3.5) -> (7.1571, 3.5)
  line L24 (7.1571, 3.5) -> (7.1571, 1.5)
  line L25 (7.1571, 1.5) -> (9.3, 1.5)
  line L26 (9.3, 1.5) -> (9.3, 3.5)
  line L27 (9.3, 3.5) -> (15.3071, 3.5)
  line L28 (15.3071, 3.5) -> (15.3071, 1.5)
  line L29 (15.3071, 1.5) -> (17.45, 1.5)
  line L30 (17.45, 1.5) -> (17.45, 3.5)
  line L31 (17.45, 3.5) -> (23.4571, 3.5)
  line L32 (23.4571, 3.5) -> (23.4571, 1.5)
  line L33 (23.4571, 1.5) -> (25.6, 1.5)
  line L34 (25.6, 1.5) -> (25.6, 3.5)
  line L35 (25.6, 3.5) -> (32.9, 3.5)
  line L36 (32.9, 3.5) -> (32.9, -1)
  line L37 (32.9, -1) -> (-32.9, -1)
  line L38 (-32.9, -1) -> (-32.9, 3.5)
  line L39 (-32.9, 3.5) -> (-25.4429, 3.5)
  line L40 (34.9, -1) -> (34.9, 3.8)
  line L41 (-34.9, 3.8) -> (-34.9, -1)
  line L42 (-34.9, -1) -> (34.9, -1)
  line L43 (34.9, 3.8) -> (-34.9, 3.8)
  constraint horizontal L3
  constraint vertical L4
  constraint horizontal L5
  constraint vertical L6
extrude "Extrude12" cut sketch "Sketch9" against normal blind 2 contours L3 L4 L5 L6 L36 L37 L42
sketch "Sketch10" plane through (-35.9, 0, 0) normal (-1, 0, 0) x (0, -1, 0)
  line L0 (34.9, 3.5) -> (34.9, 3.8)
  line L1 (34.9, 3.8) -> (-34.9, 3.8)
  line L2 (-34.9, 3.8) -> (-34.9, 3.5)
  line L3 (22.4, 3.5) -> (22.4, 1.5)
  line L4 (22.4, 1.5) -> (24.5429, 1.5)
  line L5 (24.5429, 1.5) -> (24.5429, 3.5)
  line L6 (24.5429, 3.5) -> (32.9, 3.5)
  line L7 (32.9, 3.5) -> (32.9, -1)
  line L8 (32.9, -1) -> (-32.9, -1)
  line L9 (-32.9, -1) -> (-32.9, 3.5)
  line L10 (-32.9, 3.5) -> (-25.6, 3.5)
  line L11 (-25.6, 3.5) -> (-25.6, 1.5)
  line L12 (-25.6, 1.5) -> (-23.4571, 1.5)
  line L13 (-23.4571, 1.5) -> (-23.4571, 3.5)
  line L14 (-23.4571, 3.5) -> (-17.6, 3.5)
  line L15 (-17.6, 3.5) -> (-17.6, 1.5)
  line L16 (-17.6, 1.5) -> (-15.4571, 1.5)
  line L17 (-15.4571, 1.5) -> (-15.4571, 3.5)
  line L18 (-15.4571, 3.5) -> (-9.6, 3.5)
  line L19 (-9.6, 3.5) -> (-9.6, 1.5)
  line L20 (-9.6, 1.5) -> (-7.4571, 1.5)
  line L21 (-7.4571, 1.5) -> (-7.4571, 3.5)
  line L22 (-7.4571, 3.5) -> (-1.6, 3.5)
  line L23 (-1.6, 3.5) -> (-1.6, 1.5)
  line L24 (-1.6, 1.5) -> (0.5429, 1.5)
  line L25 (0.5429, 1.5) -> (0.5429, 3.5)
  line L26 (0.5429, 3.5) -> (6.4, 3.5)
  line L27 (6.4, 3.5) -> (6.4, 1.5)
  line L28 (6.4, 1.5) -> (8.5429, 1.5)
  line L29 (8.5429, 1.5) -> (8.5429, 3.5)
  line L30 (8.5429, 3.5) -> (14.4, 3.5)
  line L31 (14.4, 3.5) -> (14.4, 1.5)
  line L32 (14.4, 1.5) -> (16.5429, 1.5)
  line L33 (16.5429, 1.5) -> (16.5429, 3.5)
  line L34 (16.5429, 3.5) -> (22.4, 3.5)
  line L35 (32.9, -1) -> (24.5429, -1)
  line L36 (24.5429, -1) -> (24.5429, 1.5)
  line L37 (24.5429, 1.5) -> (32.9, 1.5)
  line L38 (32.9, 1.5) -> (32.9, -1)
  line L39 (-34.9, 3.5) -> (34.9, 3.5)
  line L40 (34.9, -1) -> (34.9, 3.8)
  line L41 (-34.9, 3.8) -> (-34.9, -1)
  line L42 (-34.9, -1) -> (34.9, -1)
  line L43 (34.9, 3.8) -> (-34.9, 3.8)
  constraint horizontal L35
  constraint vertical L36
  constraint horizontal L37
  constraint vertical L38
  constraint coincident L4.end L5.start
  constraint coincident L7.end L8.start
extrude "Extrude13" cut sketch "Sketch10" against normal blind 2 contours L7 L8 L35 L36 L37 L38 L42
sketch "Sketch11" plane through (-26.6, 0, 0) normal (-1, 0, 0) x (0, -1, 0)
  line L0 (25.4429, 1.5) -> (32.9, 1.5)
  line L1 (30.9214, 1.5) -> (27.4214, 1.5)
  line L2 (27.4214, 1.5) -> (27.4214, 2.7)
  line L3 (27.4214, 2.7) -> (30.9214, 2.7)
  line L4 (30.9214, 2.7) -> (30.9214, 1.5)
  line L5 (17.2929, 3.5) -> (17.2929, 1.5)
  line L6 (17.2929, 1.5) -> (23.3, 1.5)
  line L7 (15.15, 1.5) -> (15.15, 3.5)
  line L8 (9.1429, 3.5) -> (9.1429, 1.5)
  line L9 (9.1429, 1.5) -> (15.15, 1.5)
  line L10 (7, 1.5) -> (7, 3.5)
  line L11 (0.9929, 3.5) -> (0.9929, 1.5)
  line L12 (0.9929, 1.5) -> (7, 1.5)
  line L13 (-1.15, 1.5) -> (-1.15, 3.5)
  line L14 (-7.1571, 3.5) -> (-7.1571, 1.5)
  line L15 (-7.1571, 1.5) -> (-1.15, 1.5)
  line L16 (-9.3, 1.5) -> (-9.3, 3.5)
  line L17 (-15.3071, 3.5) -> (-15.3071, 1.5)
  line L18 (-15.3071, 1.5) -> (-9.3, 1.5)
  line L19 (-23.4571, 1.5) -> (-17.45, 1.5)
  line L20 (-17.45, 1.5) -> (-17.45, 3.5)
  line L21 (-32.9, 3.5) -> (-32.9, 1.5)
  line L22 (-32.9, 1.5) -> (-25.6, 1.5)
  line L23 (22.0464, 1.5) -> (18.5464, 1.5)
  line L24 (22.0464, 2.7) -> (22.0464, 1.5)
  line L25 (18.5464, 1.5) -> (18.5464, 2.7)
  line L26 (18.5464, 2.7) -> (22.0464, 2.7)
  line L27 (13.8964, 1.5) -> (10.3964, 1.5)
  line L28 (13.8964, 2.7) -> (13.8964, 1.5)
  line L29 (10.3964, 1.5) -> (10.3964, 2.7)
  line L30 (10.3964, 2.7) -> (13.8964, 2.7)
  line L31 (5.7464, 1.5) -> (2.2464, 1.5)
  line L32 (5.7464, 2.7) -> (5.7464, 1.5)
  line L33 (2.2464, 1.5) -> (2.2464, 2.7)
  line L34 (2.2464, 2.7) -> (5.7464, 2.7)
  line L35 (-2.4036, 1.5) -> (-5.9036, 1.5)
  line L36 (-2.4036, 2.7) -> (-2.4036, 1.5)
  line L37 (-5.9036, 1.5) -> (-5.9036, 2.7)
  line L38 (-5.9036, 2.7) -> (-2.4036, 2.7)
  line L39 (-10.5536, 1.5) -> (-14.0536, 1.5)
  line L40 (-10.5536, 2.7) -> (-10.5536, 1.5)
  line L41 (-14.0536, 1.5) -> (-14.0536, 2.7)
  line L42 (-14.0536, 2.7) -> (-10.5536, 2.7)
  line L43 (-18.7036, 1.5) -> (-22.2036, 1.5)
  line L44 (-18.7036, 2.7) -> (-18.7036, 1.5)
  line L45 (-22.2036, 1.5) -> (-22.2036, 2.7)
  line L46 (-22.2036, 2.7) -> (-18.7036, 2.7)
  line L47 (-27.5, 1.5) -> (-31, 1.5)
  line L48 (-27.5, 2.7) -> (-27.5, 1.5)
  line L49 (-31, 1.5) -> (-31, 2.7)
  line L50 (-31, 2.7) -> (-27.5, 2.7)
  line L51 (-23.4571, 3.5) -> (-23.4571, 1.5)
  line L52 (-25.6, 1.5) -> (-25.6, 3.5)
  line L53 (25.4429, 3.5) -> (25.4429, 1.5)
  line L54 (32.9, 1.5) -> (32.9, 3.5)
  line L55 (23.3, 1.5) -> (23.3, 3.5)
  line L56 (32.9, 3.5) -> (25.4429, 3.5)
  line L57 (23.3, 3.5) -> (17.2929, 3.5)
  line L58 (15.15, 3.5) -> (9.1429, 3.5)
  line L59 (7, 3.5) -> (0.9929, 3.5)
  line L60 (-1.15, 3.5) -> (-7.1571, 3.5)
  line L61 (-9.3, 3.5) -> (-15.3071, 3.5)
  line L62 (-17.45, 3.5) -> (-23.4571, 3.5)
  line L63 (-25.6, 3.5) -> (-32.9, 3.5)
  dimension "d67" = 3.5
  dimension "d68" = 1.2
  dimension "d75" = 3.5
  dimension "d76" = 1.2
  dimension "d77" = 3.5
  dimension "d78" = 1.2
  dimension "d79" = 3.5
  dimension "d80" = 1.2
  dimension "d81" = 3.5
  dimension "d82" = 1.2
  dimension "d83" = 3.5
  dimension "d84" = 1.2
  dimension "d85" = 3.5
  dimension "d86" = 1.2
  dimension "d87" = 3.5
  dimension "d88" = 1.2
  constraint horizontal L1
  constraint vertical L2
  constraint horizontal L3
  constraint vertical L4
  constraint midpoint L0 L1
  constraint horizontal L23
  constraint vertical L25
  constraint horizontal L26
  constraint vertical L24
  constraint horizontal L27
  constraint vertical L29
  constraint horizontal L30
  constraint vertical L28
  constraint horizontal L31
  constraint vertical L33
  constraint horizontal L34
  constraint vertical L32
  constraint horizontal L35
  constraint vertical L37
  constraint horizontal L38
  constraint vertical L36
  constraint horizontal L39
  constraint vertical L41
  constraint horizontal L42
  constraint vertical L40
  constraint horizontal L43
  constraint vertical L45
  constraint horizontal L46
  constraint vertical L44
  constraint horizontal L47
  constraint vertical L49
  constraint horizontal L50
  constraint vertical L48
  constraint midpoint L6 L23
  constraint midpoint L9 L27
  constraint midpoint L12 L31
  constraint midpoint L15 L35
  constraint midpoint L18 L39
  constraint midpoint L19 L43
  constraint midpoint L22 L47
  measures "d67" distance of L1.start L1.end
  measures "d68" distance of L1.start L3.end
  measures "d75" distance of L23.start L23.end
  measures "d76" distance of L23.start L24.start
  measures "d77" distance of L27.start L27.end
  measures "d78" distance of L27.start L28.start
  measures "d79" distance of L31.start L31.end
  measures "d80" distance of L31.start L32.start
  measures "d81" distance of L35.start L35.end
  measures "d82" distance of L35.start L36.start
  measures "d83" distance of L39.start L39.end
  measures "d84" distance of L39.start L40.start
  measures "d85" distance of L43.start L43.end
  measures "d86" distance of L43.start L44.start
  measures "d87" distance of L47.start L47.end
  measures "d88" distance of L47.start L48.start
extrude "Extrude14" cut sketch "Sketch11" against normal blind 53.5 contours L0 L1 L2 L3 L4 | L6 L23 L24 L25 L26 | L9 L27 L28 L29 L30 | L12 L31 L32 L33 L34 | L15 L35 L36 L37 L38 | L18 L39 L40 L41 L42 | L19 L43 L44 L45 L46 | L22 L47 L48 L49 L50
sketch "Sketch12" plane through (0, 0, 3.8) normal (0, 0, 1) x (-1, 0, 0)
  line L0 (35.9, -34.9) -> (35.9, 34.9)
  line L1 (35.9, 34.9) -> (-35.9, 34.9)
  line L2 (-35.9, 34.9) -> (-35.9, -34.9)
  line L3 (-35.9, -34.9) -> (35.9, -34.9)
  circle A0 centre (-15.9, 34.9) radius 1.5
  circle A1 centre (-35.9, 14.9) radius 1.5
  dimension "d93" = 3
  dimension "d94" = 3
  dimension "d95" = 20
  dimension "d96" = 20
  constraint coincident L1 A0.centre
  constraint coincident L2 A1.centre
  measures "d93" diameter of A0
  measures "d94" diameter of A1
  measures "d95" distance of L2 A0.centre
  measures "d96" distance of L1 A1.centre
extrude "Extrude16" add sketch "Sketch12" against normal blind 4.8 contours L1 A0 picked at (-16.0113, 36.0676)
extrude "Extrude17" add sketch "Sketch12" against normal blind 4.8 contours L2 A1 picked at (-36.7784, 15.323)
ref_plane "WorkPlane1" through (0, 0, 1.4) normal (-1, 0, 0) x (0, -1, 0)
ref_plane "WorkPlane2" through (0, 0, 1.4) normal (0, 1, 0) x (-1, 0, 0)
mirror "Mirror1" about plane through (0, 0, 1.4) normal (0, 1, 0) of "Extrude16"
mirror "Mirror2" about plane through (0, 0, 1.4) normal (-1, 0, 0) of "Extrude16", "Mirror1"
mirror "Mirror3" about plane through (0, 0, 1.4) normal (0, 1, 0) of "Extrude17"
mirror "Mirror4" about plane through (0, 0, 1.4) normal (-1, 0, 0) of "Extrude17", "Mirror3"
equation "d27 = d26"
equation "d29 = d28"
equation "d75 = d67"
equation "d77 = d75"
equation "d79 = d77"
equation "d81 = d79"
equation "d83 = d81"
equation "d85 = d83"
equation "d87 = d85"
